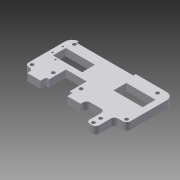
# Autodesk Inventor part: XcrRight_a
Saved by Autodesk Inventor 2013 (Build 170138000, 138)
## iProperties
Created: 2015-01-14
Part Number: XcrRight_a
Material: Generic
Document SubType Name: Modeling
Designer: dzban
Density: 1 g/cm^3
Author: dzban
Autodesk Inventor part; units mm, degrees
ref_plane "YZ Plane" through (0, 0, 0) normal (1, 0, 0) x (0, 1, 0)
ref_plane "XZ Plane" through (0, 0, 0) normal (0, 1, 0) x (-1, 0, 0)
ref_plane "XY Plane" through (0, 0, 0) normal (0, 0, 1) x (1, 0, 0)
sketch "Sketch1" plane through (0, 0, 0) normal (0, 0, 1) x (1, 0, 0)
  line L0 (-34.1796, -8.5097) -> (-34.1796, 5.4903)
  line L1 (-34.1796, 5.4903) -> (-17.1796, 5.4903)
  line L2 (-17.1796, 5.4903) -> (-17.1796, -8.5097)
  line L3 (-14.6796, -8.5097) -> (-17.1796, -8.5097)
  line L4 (-14.6796, -13.0097) -> (-14.6796, -8.5097)
  line L5 (-3.6796, -13.0097) -> (-14.6796, -13.0097)
  line L6 (-3.6796, -11.0097) -> (-3.6796, -13.0097)
  arc A0 (-0.6796, -8.0097) -> (-3.6796, -11.0097) centre (-0.6796, -11.0097) ccw
  line L7 (8.3204, -8.0097) -> (-0.6796, -8.0097)
  arc A1 (11.3204, -11.0097) -> (8.3204, -8.0097) centre (8.3204, -11.0097) ccw
  line L8 (11.3204, -20.4968) -> (11.3204, -11.0097)
  arc A2 (11.3204, -20.4968) -> (14.3204, -23.4968) centre (14.3204, -20.4968) ccw
  line L9 (16.3204, -23.4968) -> (14.3204, -23.4968)
  arc A3 (16.3204, -23.4968) -> (19.3204, -20.4968) centre (16.3204, -20.4968) ccw
  line L10 (19.3204, -11.0097) -> (19.3204, -20.4968)
  arc A4 (22.3204, -8.0097) -> (19.3204, -11.0097) centre (22.3204, -11.0097) ccw
  line L11 (26.3204, -8.0097) -> (22.3204, -8.0097)
  arc A5 (26.3204, -8.0097) -> (29.3204, -5.0097) centre (26.3204, -5.0097) ccw
  line L12 (29.3204, 24.9903) -> (29.3204, -5.0097)
  arc A6 (29.3204, 24.9903) -> (23.3204, 30.9903) centre (23.3204, 24.9903) ccw
  line L13 (-2.1796, 30.9903) -> (23.3204, 30.9903)
  line L14 (-2.1796, 28.9903) -> (-2.1796, 30.9903)
  line L15 (-49.1796, 28.9903) -> (-2.1796, 28.9903)
  line L16 (-49.1796, 30.9903) -> (-49.1796, 28.9903)
  arc A7 (-49.1796, 30.9903) -> (-54.6796, 25.0112) centre (-48.6796, 25.0112) ccw
  line L17 (-54.6796, -5.0097) -> (-54.6796, 25.0112)
  arc A8 (-54.6796, -5.0097) -> (-51.6796, -8.0097) centre (-51.6796, -5.0097) ccw
  line L18 (-50.6796, -8.0097) -> (-51.6796, -8.0097)
  arc A9 (-47.6796, -11.0097) -> (-50.6796, -8.0097) centre (-50.6796, -11.0097) ccw
  line L19 (-47.6796, -13.0097) -> (-47.6796, -11.0097)
  line L20 (-36.6796, -13.0097) -> (-47.6796, -13.0097)
  line L21 (-36.6796, -8.5097) -> (-36.6796, -13.0097)
  line L22 (-34.1796, -8.5097) -> (-36.6796, -8.5097)
  circle A10 centre (15.0119, -15.1214) radius 1.5
  circle A11 centre (15.0119, -21.1214) radius 1.5
  circle A12 centre (-51.9296, 20.6159) radius 0.75
  circle A13 centre (-51.9296, 12.1159) radius 0.75
  circle A14 centre (-45.6796, 8.2799) radius 0.75
  circle A15 centre (-48.6796, 26.9903) radius 1.5
  circle A16 centre (26.3204, -5.0097) radius 1.5
  circle A17 centre (-14.1796, -2.0097) radius 1.5
  circle A18 centre (-51.6796, -5.0097) radius 1.5
  circle A19 centre (20.3204, 26.4903) radius 1.5
  circle A20 centre (-37.1796, -2.0097) radius 1.5
  line L23 (-49.6796, 10.1903) -> (-49.6796, 20.7903)
  line L24 (-49.6796, 20.7903) -> (-25.6796, 20.7903)
  line L25 (-25.6796, 20.7903) -> (-25.6796, 10.1903)
  line L26 (-25.6796, 10.1903) -> (-49.6796, 10.1903)
  line L27 (0.3204, 20.7903) -> (24.3204, 20.7903)
  line L28 (24.3204, 20.7903) -> (24.3204, 10.1903)
  line L29 (24.3204, 10.1903) -> (0.3204, 10.1903)
  line L30 (0.3204, 10.1903) -> (0.3204, 20.7903)
  point P0 (0, 0)
  point P1 (0, 0)
  constraints: 62 end point, 21 centre point, 20 point on circle
extrude "Extrusion1" add sketch "Sketch1" along normal blind 6
body "Solid1"
